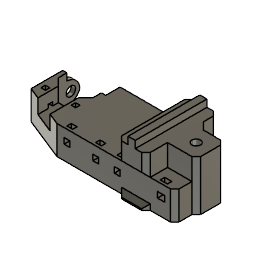
tripple leg for chain y (Autodesk Fusion 360 design; units mm, degrees)
Autodesk Fusion 360 part; units mm, degrees
sketch "Szkic1" plane through (0, 0, 0) normal (0, 0, 1) x (1, 0, 0)
  line L0 (-20, 25) -> (-20, -25)
  line L1 (-20, -25) -> (0, -25)
  line L2 (0, -25) -> (0, 25)
  line L3 (0, 25) -> (-20, 25)
  line L4 (0, 10) -> (0, -10)
  line L5 (0, -10) -> (20, -10)
  line L6 (20, -10) -> (20, 10)
  line L7 (20, 10) -> (0, 10)
  circle A0 centre (10, 0) radius 3
  circle A1 centre (10, 0) radius 5.5
  line L8 (-12.5, 25) -> (-7.5, 25)
  line L9 (-7.5, 25) -> (-7.5, -25)
  line L10 (-7.5, -25) -> (-12.5, -25)
  line L11 (-12.5, -25) -> (-12.5, 25)
  dimension "d1" = 6
  dimension "d2" = 11
  constraint perpendicular L0 L1
  constraint parallel L0 L2
  constraint parallel L1 L3
  constraint vertical L0
  constraint perpendicular L4 L5
  constraint parallel L4 L6
  constraint parallel L5 L7
  constraint coincident L2 L4.end
  constraint parallel L2 L4
  constraint concentric A0 A1
  constraint perpendicular L8 L9
  constraint parallel L8 L10
  constraint parallel L9 L11
  constraint coincident L3 L8.end
  constraint coincident L3 L8.start
  measures "d1" diameter of A0
  measures "d2" diameter of A1
extrude "Wyciągnięcie proste1" add sketch "Szkic1" against normal blind 25 contours L0 L1 L3 L11 | L1 L3 L8 L9 L10 L11 | L1 L2 L3 L4 L9 | L2 L4 L5 L6 L7
extrude "Wyciągnięcie proste2" add sketch "Szkic1" against normal blind 4.2 contours A0 | A1
extrude "Wyciągnięcie proste3" cut sketch "Szkic1" against normal blind 4 contours A0
extrude "Wyciągnięcie proste4" add sketch "Szkic1" along normal blind 5 contours L1 L3 L8 L9 L10 L11
chamfer "Fazowanie1" distance 5 angle 45 1 edges at (0, -10, -12.5) tangent chain off
chamfer "Fazowanie2" distance 5 angle 45 1 edges at (0, 10, -12.5) tangent chain off
chamfer "Fazowanie3" distance 3 angle 45 6 edges at (20, 10, -12.5) (20, -10, -12.5) (0, 25, -12.5) (-20, 25, -12.5) (-20, -25, -12.5) (0, -25, -12.5) tangent chain off
chamfer "Fazowanie4" distance 1 angle 45 1 faces at (-11.8333, 0, -25) tangent chain off
delete_face "Usuń powierzchnię1" 1 faces at (16.159, -0.3074, -24.6667)
delete_face "Usuń powierzchnię2" 1 faces at (-1.3333, 22.8619, -24.3333)
delete_face "Usuń powierzchnię3" 1 faces at (-0.6667, 19.8619, -24.6667)
delete_face "Usuń powierzchnię4" 1 faces at (1.6667, 12.8619, -24.3333)
delete_face "Usuń powierzchnię5" 1 faces at (9.3333, 9.6667, -24.3333)
delete_face "Usuń powierzchnię6" 1 faces at (19.6667, -2.1953, -24.3333)
delete_face "Usuń powierzchnię7" 1 faces at (-0.3333, -19.5286, -24.3333)
delete_face "Usuń powierzchnię8" 1 faces at (17.5286, 8.5286, -24.6667)
delete_face "Usuń powierzchnię9" 1 faces at (-7.1953, 24.3333, -24.6667)
delete_face "Usuń powierzchnię10" 1 faces at (-17.1953, 23.8619, -24.6667)
delete_face "Usuń powierzchnię11" 1 faces at (-7.8047, -24.6667, -24.3333)
delete_face "Usuń powierzchnię12" 1 faces at (-17.1953, -23.8619, -24.6667)
delete_face "Usuń powierzchnię13" 1 faces at (-19.3333, -7.3333, -24.6667)
delete_face "Usuń powierzchnię14" 1 faces at (18.8619, -7.1953, -24.6667)
delete_face "Usuń powierzchnię15" 1 faces at (13.1953, -9.3333, -24.6667)
delete_face "Usuń powierzchnię16" 1 faces at (2.8619, -11.6667, -24.3333)
delete_face "Usuń powierzchnię17" 1 faces at (-2.4714, -23.5286, -24.6667)
extrude "Wyciągnięcie proste5" add 1 faces at (-11.8333, 0, -25) along direction (0, 0, -1) blind 10
extrude "Wyciągnięcie proste6" add 1 faces at (-20, -7.3333, -23.3333) along direction (-1, 0, 0) blind 45
sketch "Szkic2" plane through (0, 0, 0) normal (0, 0, 1) x (-1, 0, 0)
  line L0 (20, 22) -> (17, 25)
  line L1 (17, 25) -> (12.5, 25)
  line L2 (12.5, 25) -> (12.5, -25)
  line L3 (12.5, -25) -> (17, -25)
  line L4 (17, -25) -> (20, -22)
  line L5 (20, -22) -> (65, -22)
  line L6 (65, -22) -> (65, 22)
  line L7 (65, 22) -> (20, 22)
  line L8 (20, -22) -> (20, 22)
  line L9 (20, 22) -> (65, 22)
  line L10 (65, 22) -> (65, -22)
  line L11 (65, -22) -> (20, -22)
  constraint perpendicular L8 L9
  constraint parallel L8 L10
  constraint parallel L9 L11
  constraint coincident L0.start L7.end
  constraint perpendicular L7 L8
  constraint coincident L4.end L5.start
extrude "Wyciągnięcie proste7" cut sketch "Szkic2" against normal blind 15 contours L5 L6 L7 L8 L9 L10 L11
extrude "Wyciągnięcie proste8" cut 1 faces at (-35, 7.3333, -15) along direction (0, 0, -1) blind 5
sketch "Szkic3" plane through (0, 0, -20) normal (0, 0, 1) x (-1, 0, 0)
  line L0 (65, -22) -> (65, 22)
  line L1 (65, 22) -> (20, 22)
  line L2 (20, 22) -> (20, -22)
  line L3 (20, -22) -> (65, -22)
  line L4 (87, -1) -> (92, -6)
  line L5 (95, -21.25) -> (95, -2)
  line L6 (94, -1) -> (87, -1)
  line L7 (68, -21.25) -> (65, -21.25)
  line L8 (65, -1) -> (68, -1)
  line L9 (92, -21.25) -> (92, -1)
  line L10 (92, -1) -> (95, -1)
  line L11 (95, -21.25) -> (92, -21.25)
  line L12 (65, -21.25) -> (65, -1)
  line L13 (92, -6) -> (92, -21.25)
  line L14 (95, -1) -> (95, -21.25)
  line L15 (92, -21.25) -> (95, -21.25)
  line L16 (68, -1) -> (68, -21.25)
  line L17 (95, -1) -> (65, -1)
  line L18 (65, -1) -> (65, 10)
  line L19 (65, 10) -> (95, 10)
  line L20 (95, 10) -> (95, -1)
  line L21 (73, -1) -> (68, -6)
  constraint perpendicular L9 L11
  constraint parallel L10 L11
  constraint parallel L9 L14
  constraint coincident L9.start L11.end
  constraint perpendicular L11 L13
  constraint coincident L5.start L11.start
  constraint perpendicular L7 L12
  constraint parallel L7 L8
  constraint parallel L12 L16
  constraint perpendicular L17 L18
  constraint parallel L17 L19
  constraint parallel L18 L20
  constraint perpendicular L0 L17
  constraint coincident L17 L21.start
  constraint coincident L16 L21.end
extrude "Wyciągnięcie proste9" add sketch "Szkic3" against normal blind 15 contours L0 L7 L8 L12 L16 L17 | L0 L6 L8 L10 L17 L18 L19 L20 | L16 L17 L21 | L5 L6 L9 L10 L11 L13 L14 L15 L17 | L4 L6 L9 L17
extrude "Wyciągnięcie proste10" add 1 faces at (-67, 21.25, -25) along direction (0, 1, 0) blind 0.75
extrude "Wyciągnięcie proste11" add 1 faces at (-94, 21.25, -25) along direction (0, 1, 0) blind 0.75
sketch "Szkic4" plane through (-68, 0, 0) normal (-1, 0, 0) x (0, -1, 0)
  line L0 (-6, -20) -> (-22, -20)
  line L1 (-22, -20) -> (-22, -35)
  line L2 (-22, -35) -> (-6, -35)
  line L3 (-6, -35) -> (-6, -20)
  line L4 (-22, -27.5) -> (-18, -27.5)
  circle A0 centre (-14.75, -27.5) radius 3.25
  dimension "d29" = 6.5
  constraint midpoint L1 L4.start
  constraint perpendicular L1 L4
  constraint coincident L4.end A0
  measures "d29" diameter of A0
extrude "Wyciągnięcie proste12" cut sketch "Szkic4" along normal blind 40 contours A0
extrude "Wyciągnięcie proste13" cut sketch "Szkic4" against normal blind 3 contours A0
sketch "Szkic5" plane through (0, 22, 0) normal (0, 1, 0) x (-1, 0, 0)
  line L0 (68, -20) -> (20, -20)
  line L1 (20, -20) -> (20, -35)
  line L2 (20, -35) -> (68, -35)
  line L3 (68, -35) -> (68, -20)
  line L4 (68, -20) -> (68, -35)
  line L5 (68, -35) -> (65, -35)
  line L6 (65, -35) -> (65, -20)
  line L7 (65, -20) -> (68, -20)
  line L8 (92, -20) -> (95, -20)
  line L9 (95, -20) -> (95, -35)
  line L10 (95, -35) -> (92, -35)
  line L11 (92, -35) -> (92, -20)
  constraint perpendicular L4 L5
  constraint parallel L4 L6
  constraint parallel L5 L7
  constraint coincident L2.end L3.start
  constraint perpendicular L2 L4
  constraint coincident L0.start L3.end
  constraint perpendicular L8 L9
  constraint parallel L8 L10
  constraint parallel L9 L11
  constraint horizontal L8
extrude "Wyciągnięcie proste14" cut sketch "Szkic5" against normal blind 1 contours L0 L2 L3 L4 L5 L6 L7 | L8 L9 L10 L11
fillet "Zaokrąglenie1" radius 9 1 edges at (-66.5, 21, -20)
fillet "Zaokrąglenie2" radius 9 1 edges at (-93.5, 21, -20)
fillet "Zaokrąglenie3" radius 9 2 edges at (-93.5, 21, -35) (-66.5, 21, -35)
chamfer "Fazowanie5" distance 12 distance2 30 1 edges at (-65, -10, -27.5) measured on face at (-65, -18, -30) tangent chain off
chamfer "Fazowanie6" distance 7 distance2 7 1 edges at (-20, 0, -20) measured on face at (-20, 7.3333, -6.6667) tangent chain off
delete_face "Usuń powierzchnię18" 1 faces at (-24.6667, 7.3333, -17.6667)
extrude "Wyciągnięcie proste15" add 1 faces at (-35, 4, -20) along direction (0, 0, 1) blind 5
sketch "Szkic6" plane through (0, 1, 0) normal (0, 1, 0) x (-1, 0, 0)
  line L0 (73, -15) -> (73, -35)
  line L1 (73, -35) -> (87, -35)
  line L2 (87, -35) -> (87, -15)
  line L3 (87, -15) -> (73, -15)
  line L4 (73, -15) -> (87, -15)
  line L5 (87, -15) -> (87, -25)
  line L6 (87, -25) -> (73, -25)
  line L7 (73, -25) -> (73, -15)
  constraint perpendicular L4 L5
  constraint parallel L4 L6
  constraint parallel L5 L7
  constraint coincident L2.end L3.start
  constraint perpendicular L2 L4
  constraint coincident L0.start L3.end
extrude "Wyciągnięcie proste16" cut sketch "Szkic6" against normal blind 47 contours L0 L2 L3 L4 L5 L6 L7
sketch "Szkic7" plane through (0, 0, -15) normal (0, 0, 1) x (-1, 0, 0)
  line L0 (73, -1) -> (73, 18.8)
  line L1 (73, 18.8) -> (65, 22)
  line L2 (65, 22) -> (20, 22)
  line L3 (20, 22) -> (20, -22)
  line L4 (20, -22) -> (65, -22)
  line L5 (65, -22) -> (65, -12)
  line L6 (65, -12) -> (68, -12)
  line L7 (68, -12) -> (68, -6)
  line L8 (68, -6) -> (73, -1)
  line L9 (89, 3) -> (92, 3)
  line L10 (92, 3) -> (92, 6)
  line L11 (92, 6) -> (89, 6)
  line L12 (89, 6) -> (89, 3)
  line L13 (71, 3) -> (68, 3)
  line L14 (68, 3) -> (68, 6)
  line L15 (68, 6) -> (71, 6)
  line L16 (71, 6) -> (71, 3)
  line L17 (60, 20) -> (56, 20)
  line L18 (56, 20) -> (56, 17)
  line L19 (56, 17) -> (60, 17)
  line L20 (60, 17) -> (60, 20)
  line L21 (40, 17) -> (36, 17)
  line L22 (36, 17) -> (36, 20)
  line L23 (36, 20) -> (40, 20)
  line L24 (40, 20) -> (40, 17)
  line L25 (25, 17) -> (21, 17)
  line L26 (21, 17) -> (21, 20)
  line L27 (21, 20) -> (25, 20)
  line L28 (25, 20) -> (25, 17)
  constraint perpendicular L9 L10
  constraint parallel L9 L11
  constraint parallel L10 L12
  constraint horizontal L9
  constraint perpendicular L13 L14
  constraint parallel L13 L15
  constraint parallel L14 L16
  constraint horizontal L13
  constraint perpendicular L17 L18
  constraint parallel L17 L19
  constraint parallel L18 L20
  constraint horizontal L17
  constraint perpendicular L21 L22
  constraint parallel L21 L23
  constraint parallel L22 L24
  constraint horizontal L21
  constraint perpendicular L25 L26
  constraint parallel L25 L27
  constraint parallel L26 L28
  constraint horizontal L25
extrude "Wyciągnięcie proste17" cut sketch "Szkic7" against normal blind 10 contours L9 L10 L11 L12 | L13 L14 L15 L16 | L17 L18 L19 L20 | L21 L22 L23 L24 | L25 L26 L27 L28
sketch "Szkic8" plane through (0, -22, 0) normal (0, -1, 0) x (1, 0, 0)
  line L0 (-65, -15) -> (-65, -35)
  line L1 (-65, -35) -> (-20, -35)
  line L2 (-20, -35) -> (-20, -15)
  line L3 (-20, -15) -> (-65, -15)
  line L4 (-60, -15) -> (-56, -15)
  line L5 (-56, -15) -> (-56, -25)
  line L6 (-56, -25) -> (-60, -25)
  line L7 (-60, -25) -> (-60, -15)
  line L8 (-60, -21) -> (-21, -21)
  line L9 (-21, -21) -> (-21, -25)
  line L10 (-21, -25) -> (-25, -25)
  line L11 (-25, -25) -> (-25, -21)
  line L12 (-36, -21) -> (-36, -25)
  line L13 (-36, -25) -> (-40, -25)
  line L14 (-40, -25) -> (-40, -21)
  dimension "d52" = 10
  constraint perpendicular L4 L5
  constraint parallel L4 L6
  constraint parallel L5 L7
  constraint coincident L3 L4.end
  constraint coincident L3 L4.start
  constraint coincident L7 L8.start
  constraint perpendicular L7 L8
  constraint perpendicular L8 L9
  constraint perpendicular L9 L10
  constraint coincident L8 L11.end
  constraint perpendicular L8 L11
  constraint coincident L8 L12.start
  constraint perpendicular L8 L12
  constraint perpendicular L12 L13
  constraint coincident L8 L14.end
  constraint perpendicular L8 L14
  measures "d52" distance of L4.start L6.end
extrude "Wyciągnięcie proste18" cut sketch "Szkic8" against normal blind 4 contours L5 L6 L7 L8 | L8 L12 L13 L14 | L8 L9 L10 L11
sketch "Szkic9" plane through (-73, 0, 0) normal (-1, 0, 0) x (0, -1, 0)
  line L0 (18.8, -25) -> (18.8, -15)
  line L1 (18.8, -15) -> (-1, -15)
  line L2 (-1, -15) -> (-1, -25)
  line L3 (-1, -25) -> (18.8, -25)
  line L4 (3, -15) -> (6, -15)
  line L5 (6, -15) -> (6, -25)
  line L6 (6, -25) -> (3, -25)
  line L7 (3, -25) -> (3, -15)
  line L8 (3, -22.5) -> (6, -22.5)
  dimension "d55" = 10
  constraint perpendicular L4 L5
  constraint parallel L4 L6
  constraint parallel L5 L7
  constraint coincident L1 L4.end
  constraint coincident L1 L4.start
  constraint coincident L7 L8.start
  constraint perpendicular L7 L8
  measures "d55" distance of L4.start L6.end
extrude "Wyciągnięcie proste19" cut sketch "Szkic9" against normal blind 3 contours L3 L5 L6 L7 L8
extrude "Wyciągnięcie proste20" cut sketch "Szkic9" along normal blind 18 contours L3 L5 L6 L7 L8
chamfer "Fazowanie7" distance 1 distance2 2 1 edges at (-89, -4.5, -22.5) measured on face at (-89, -5, -17.5) tangent chain off
chamfer "Fazowanie8" distance 1 distance2 1 1 edges at (-71, -4.5, -22.5) measured on face at (-71, -5, -17.5) tangent chain off
chamfer "Fazowanie9" distance 1 distance2 1 1 edges at (-68, -4.5, -25) measured on face at (-68, -4, -18.3333) tangent chain off
chamfer "Fazowanie10" distance 1 distance2 1 1 edges at (-92, -4.5, -25) measured on face at (-92, -4, -18.3333) tangent chain off
chamfer "Fazowanie11" distance 1 distance2 1 3 edges at (-58, -17, -25) (-38, -17, -25) (-23, -17, -25) measured on face at (-57.3333, -17, -18.3333) measured on face at (-38.6667, -17, -18.3333) measured on face at (-23.6667, -17, -18.3333) tangent chain off
chamfer "Fazowanie12" distance 1 distance2 1 3 edges at (-58, -20, -21) (-38, -20, -21) (-23, -20, -21) measured on face at (-58.6667, -20, -17) measured on face at (-37.3333, -20, -17) measured on face at (-22.3333, -20, -17) tangent chain off
delete_face "Usuń powierzchnię19" 1 faces at (1.6667, -13.3333, -11.6667)
sketch "Szkic10" plane through (0, 0, 0) normal (1, 0, 0) x (0, 1, 0)
  line L0 (-22, -35) -> (-10, -35)
  line L1 (-10, -35) -> (-10, 0)
  line L2 (-10, 0) -> (-22, 0)
  line L3 (-22, 0) -> (-22, -35)
  line L4 (-10, -35) -> (-10, -15)
  line L5 (-10, -15) -> (-22, -15)
  line L6 (-22, -15) -> (-22, -35)
  line L7 (-22, -35) -> (-10, -35)
  constraint perpendicular L4 L5
  constraint parallel L4 L6
  constraint parallel L5 L7
  constraint coincident L1 L4.end
  constraint perpendicular L0 L4
  constraint coincident L0.end L1.start
extrude "Wyciągnięcie proste21" add sketch "Szkic10" along normal blind 17 contours L0 L1 L3 L4 L5 L6 L7
sketch "Szkic11" plane through (0, 0, -15) normal (0, 0, 1) x (-1, 0, 0)
  line L0 (0, 10) -> (0, 22)
  line L1 (0, 22) -> (-17, 22)
  line L2 (-17, 22) -> (-17, 10)
  line L3 (-17, 10) -> (0, 10)
  line L4 (-5, 20) -> (-10, 20)
  line L5 (-10, 20) -> (-10, 17)
  line L6 (-10, 17) -> (-5, 17)
  line L7 (-5, 17) -> (-5, 20)
  constraint perpendicular L4 L5
  constraint parallel L4 L6
  constraint parallel L5 L7
  constraint horizontal L4
extrude "Wyciągnięcie proste22" cut sketch "Szkic11" against normal blind 10 contours L4 L5 L6 L7
sketch "Szkic12" plane through (0, -22, 0) normal (0, -1, 0) x (1, 0, 0)
  line L0 (0, -15) -> (0, -35)
  line L1 (0, -35) -> (17, -35)
  line L2 (17, -35) -> (17, -15)
  line L3 (17, -15) -> (0, -15)
  line L4 (5, -15) -> (10, -15)
  line L5 (10, -15) -> (10, -25)
  line L6 (10, -25) -> (5, -25)
  line L7 (5, -25) -> (5, -15)
  line L8 (5, -21) -> (10, -21)
  dimension "d76" = 10
  constraint perpendicular L4 L5
  constraint parallel L4 L6
  constraint parallel L5 L7
  constraint coincident L3 L4.end
  constraint coincident L3 L4.start
  constraint coincident L7 L8.start
  constraint coincident L5 L8.end
  constraint perpendicular L5 L8
  measures "d76" distance of L4.start L6.end
extrude "Wyciągnięcie proste23" cut sketch "Szkic12" against normal blind 3 contours L5 L6 L7 L8
chamfer "Fazowanie13" distance 1 distance2 1 1 edges at (7.5, -17, -25) measured on face at (8.3333, -17, -18.3333) tangent chain off
chamfer "Fazowanie14" distance 1 distance2 1 1 edges at (7.5, -20, -21) measured on face at (6.6667, -20, -17) tangent chain off
sketch "Szkic13" plane through (0, -25, 0) normal (0, -1, 0) x (1, 0, 0)
  line L0 (-3, -35) -> (-3, 0)
  line L1 (-3, 0) -> (-7.5, 0)
  line L2 (-7.5, 0) -> (-7.5, 5)
  line L3 (-7.5, 5) -> (-12.5, 5)
  line L4 (-12.5, 5) -> (-12.5, 0)
  line L5 (-12.5, 0) -> (-17, 0)
  line L6 (-17, 0) -> (-17, -35)
  line L7 (-17, -35) -> (-3, -35)
  line L8 (-20, -15) -> (0, -15)
  line L9 (0, -15) -> (0, -31)
  line L10 (0, -31) -> (-20, -31)
  line L11 (-20, -31) -> (-20, -15)
  constraint perpendicular L8 L9
  constraint parallel L8 L10
  constraint parallel L9 L11
  constraint horizontal L8
extrude "Wyciągnięcie proste24" cut sketch "Szkic13" against normal blind 3 contours L0 L6 L8 L10 | L0 L8 L9 L10 | L6 L8 L10 L11
chamfer "Fazowanie15" distance 3 distance2 3 1 edges at (-10, -25, -15) measured on face at (-9.1667, -25, -10) tangent chain off
chamfer "Fazowanie16" distance 3 distance2 3 1 edges at (-10, -25, -31) measured on face at (-12.3333, -25, -32.3333) tangent chain off
chamfer "Fazowanie17" distance 3 distance2 3 1 edges at (17, -22, -25) measured on face at (17, -18, -21.6667) tangent chain off
